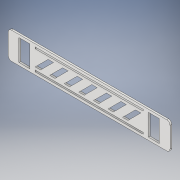
# Autodesk Inventor part: Cuerpo - LateralPrueba
Saved by Autodesk Inventor 2019 (Build 230136000, 136)
## iProperties
Created: 2020-02-14
Part Number: Cuerpo - LateralPrueba
Material: ABS Plastic
Document SubType Name: Modeling
Designer: Mafer1
Density: 1.06 g/cm^3
Appearance: Smooth - White
Mass: 36.6909 g
Surface Area: 287.559 cm^2
Volume: 34.614 cm^3
base_servo: 20.000 mm
altura_servo: 40.000 mm
agujero_servo: 2.000 mm
distancia_agujero_servo: 1.750 mm
soporte: 60.000 mm
largo_base: 200.000 mm
Author: Mafer1
Autodesk Inventor part; units mm, degrees
ref_plane "YZ Plane" through (0, 0, 0) normal (1, 0, 0) x (0, 1, 0)
ref_plane "XZ Plane" through (0, 0, 0) normal (0, 1, 0) x (-1, 0, 0)
ref_plane "XY Plane" through (0, 0, 0) normal (0, 0, 1) x (1, 0, 0)
sketch "Sketch7" plane through (0, 0, 0) normal (0, 0, 1) x (1, 0, 0)
  line L0 (0, 0) -> (300, 0)
  line L1 (300, 0) -> (300, 50)
  line L2 (300, 50) -> (0, 50)
  line L3 (0, 50) -> (0, 0)
  line L4 (50, 8) -> (250, 8)
  line L5 (250, 8) -> (250, 5)
  line L6 (250, 5) -> (50, 5)
  line L7 (50, 5) -> (50, 8)
  line L8 (150, 8) -> (150, 5) construction
  line L9 (20, 45) -> (40, 45)
  line L10 (40, 45) -> (40, 5)
  line L11 (40, 5) -> (20, 5)
  line L12 (20, 5) -> (20, 45)
  line L13 (260, 45) -> (280, 45)
  line L14 (280, 45) -> (280, 5)
  line L15 (280, 5) -> (260, 5)
  line L16 (260, 5) -> (260, 45)
  line L17 (50, 42) -> (250, 42)
  line L18 (250, 42) -> (250, 45)
  line L19 (250, 45) -> (50, 45)
  line L20 (50, 45) -> (50, 42)
  point P0 (50, 43.5)
  point P1 (50, 6.5)
  dimension "d152" = 300
  dimension "d153" = 50
  dimension "d154" = 200
  dimension "d158" = 150
  dimension "d159" = 3
  dimension "d160" = 5
  dimension "d161" = 40
  dimension "d162" = 20
  dimension "d163" = 20
  dimension "d164" = 20
  dimension "d165" = 5
  dimension "d166" = 5
  dimension "d168" = 5
  constraints: 42 end point, 10 parallel, 5 horizontal, 5 perpendicular, 4 equal length, 4 midpoint, 1 vertical alignment
  measures "d152" distance of L0.start L0.end
  measures "d153" distance of L0.end L1.end
  measures "d154" distance of L4.start L4.end
  measures "d158" distance between parallel lines of L1 L8
  measures "d159" distance between parallel lines of L6 L4
  measures "d160" distance between parallel lines of L0 L6
  measures "d161" distance of L9.end L10.end
  measures "d162" distance of L9.start L9.end
  measures "d163" distance between parallel lines of L12 L3
  measures "d164" distance between parallel lines of L14 L1
  measures "d165" distance between parallel lines of L11 L0
  measures "d166" distance between parallel lines of L0 L15
  measures "d168" distance between parallel lines of L19 L2
extrude "Extrusion7" add sketch "Sketch7" along normal blind 3.3
fillet "Fillet1" radius 6 4 edges at (0, 50, 1.65) (0, 0, 1.65) (300, 50, 1.65) (300, 0, 1.65)
sketch "Sketch9" plane through (0, 0, 3.3) normal (0, 0, 1) x (1, 0, 0)
  arc A0 (294, 0) -> (300, 6) centre (294, 6) ccw projected
  line L0 (300, 6) -> (300, 44) projected
  arc A1 (300, 44) -> (294, 50) centre (294, 44) ccw projected
  line L1 (294, 50) -> (6, 50) projected
  arc A2 (6, 50) -> (0, 44) centre (6, 44) ccw projected
  line L2 (0, 44) -> (0, 6) projected
  arc A3 (0, 6) -> (6, 0) centre (6, 6) ccw projected
  line L3 (6, 0) -> (294, 0) projected
  line L4 (280, 45) -> (280, 5) projected
  line L5 (280, 5) -> (260, 5) projected
  line L6 (260, 5) -> (260, 45) projected
  line L7 (260, 45) -> (280, 45) projected
  line L8 (40, 45) -> (40, 5) projected
  line L9 (40, 5) -> (20, 5) projected
  line L10 (20, 5) -> (20, 45) projected
  line L11 (20, 45) -> (40, 45) projected
  line L12 (50, 42) -> (50, 45) projected
  line L13 (50, 45) -> (250, 45) projected
  line L14 (250, 45) -> (250, 42) projected
  line L15 (250, 42) -> (50, 42) projected
  line L16 (250, 8) -> (250, 5) projected
  line L17 (250, 5) -> (50, 5) projected
  line L18 (50, 5) -> (50, 8) projected
  line L19 (50, 8) -> (250, 8) projected
  line L20 (50, 13) -> (74, 37)
  line L21 (74, 37) -> (84, 37)
  line L22 (84, 37) -> (60, 13)
  line L23 (60, 13) -> (50, 13)
  point P0 (0, 0)
  dimension "d172" = 45
  dimension "d173" = 10
  dimension "d175" = 5
  dimension "d176" = 5
  constraints: 8 end point, 2 parallel, 1 horizontal, 1 vertical alignment
  measures "d172" angle of L23 L22
  measures "d173" distance of L20.end L21.end
  measures "d175" distance between parallel lines of L15 L21
  measures "d176" distance between parallel lines of L19 L23
extrude "Extrusion8" cut sketch "Sketch9" against normal blind 3.3 contours L20 L21 L22 L23
pattern_linear "Rectangular Pattern1" count 7 spacing 27 along (1, 0, 0) of "Extrusion8"
equation "\"soporte\" = 60"
equation "\"largo_base\" = 200"
body "Solid2"
